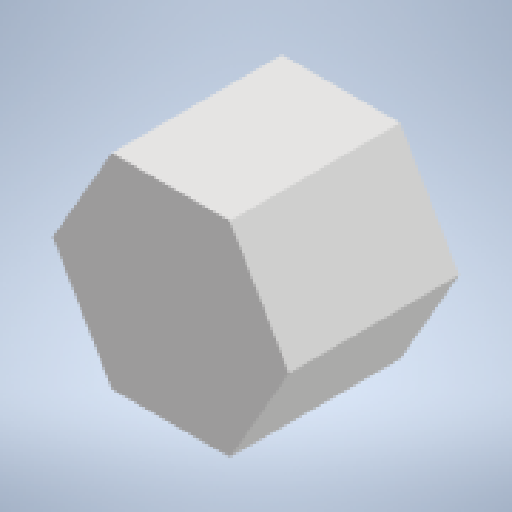
# Autodesk Inventor part: BasePGearInnerRingSupport
Saved by Autodesk Inventor 2023 (Build 270158030, 158C)
## iProperties
Created: 2024-09-26
Part Number: BasePGearInnerRingSupport
Material: Generic
Document SubType Name: Modeling
Designer: lvrectanus0
Density: 1 g/cm^3
Appearance: Default
Author: lvrectanus0
Autodesk Inventor part; units mm, degrees
ref_plane "YZ Plane" through (0, 0, 0) normal (1, 0, 0) x (0, 1, 0)
ref_plane "XZ Plane" through (0, 0, 0) normal (0, 1, 0) x (-1, 0, 0)
sketch "Sketch1" plane through (0, 0, 0) normal (0, 0, 1) x (1, 0, 0)
  circle A0 centre (0, 0) radius 15.4305 projected
  line L0 (-2.7496, 4.7625) -> (-5.4993, 0) projected
  line L1 (2.7496, 4.7625) -> (-2.7496, 4.7625) projected
  line L2 (5.4993, 0) -> (2.7496, 4.7625) projected
  line L3 (2.7496, -4.7625) -> (5.4993, 0) projected
  line L4 (-2.7496, -4.7625) -> (2.7496, -4.7625) projected
  line L5 (-5.4993, 0) -> (-2.7496, -4.7625) projected
ref_plane "Work Plane1" through (-13.7797, -13.7797, -7.9273) normal (0, 0, -1) x (0, 1, 0)
extrude "Extrusion1" add sketch "Sketch1" against normal up to surface (7.9273 mm away) contours L1 L2 L3 L4 L5 L0
body "Solid1"
